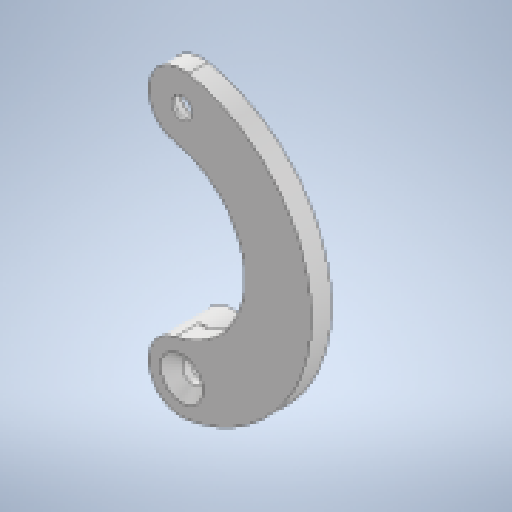
# Autodesk Inventor part: rotor_arm
Saved by Autodesk Inventor 2024 (Build 280153000, 153)
## iProperties
Created: 2025-06-26
Part Number: rotor_arm
Material: 一般
Document SubType Name: Modeling
Designer: kshau
Density: 1 g/cm^3
Appearance: 既定
Author: kshau
Autodesk Inventor part; units mm, degrees
ref_plane "YZ Plane" through (0, 0, 0) normal (1, 0, 0) x (0, 1, 0)
ref_plane "XZ Plane" through (0, 0, 0) normal (0, 1, 0) x (-1, 0, 0)
ref_plane "XY Plane" through (0, 0, 0) normal (0, 0, 1) x (1, 0, 0)
sketch "スケッチ1" plane through (0, 0, 0) normal (0, 0, 1) x (1, 0, 0)
  circle A0 centre (0, 0) radius 5
  circle A1 centre (0, 35) radius 5
  line L0 (0, 35) -> (0, 0)
  arc A2 (0.968731, -4.905258) -> (0.968731, 39.905258) centre (-3.456045, 17.5) ccw
  arc A3 (-0.968731, 4.905258) -> (-0.968731, 30.094742) centre (-3.456045, 17.5) ccw
  point P0 (0, 30)
  point P1 (0, 29.864061)
  point P2 (0, 5.135939)
  point P3 (0, 5)
  dimension "d0" = 10
  dimension "d1" = 10
  dimension "d2" = 35
  dimension "d3" = 22.838
  dimension "d4" = 12.838
  constraints: 8 point on circle, 4 centre point, 4 tangent, 2 end point, 1 coincident, 1 vertical
  measures "d0" diameter of A0
  measures "d1" diameter of A1
  measures "d2" distance of L0.end L0.start
  measures "d3" radius of A2
  measures "d4" radius of A3
extrude "押し出し1" add sketch "スケッチ1" along normal blind 3 contours A0 | A3 L0 A0 | A0 L0 A3 A1 A2 | A1 | A3 A1 L0
sketch "スケッチ2" plane through (0, 0, 0) normal (0, 0, -1) x (-1, 0, 0)
  circle A0 centre (0, 0) radius 5
  constraints: 1 centre point, 1 coincident
extrude "押し出し2" add sketch "スケッチ2" along normal blind 4.8
sketch "スケッチ3" plane through (0, 0, -4.8) normal (0, 0, -1) x (-1, 0, 0)
  circle A0 centre (0, 0) radius 3.1
  dimension "d9" = 6.2
  constraints: 1 centre point, 1 coincident
  measures "d9" diameter of A0
extrude "押し出し3" cut sketch "スケッチ3" against normal blind 5
sketch "スケッチ4" plane through (0, 0, 3) normal (0, 0, 1) x (1, 0, 0)
  circle A0 centre (0, 0) radius 3.1
  arc A1 (0.968731, 39.905258) -> (-0.968731, 30.094742) centre (0, 35) ccw
  point P0 (0, 30)
  constraints: 2 coincident
hole "穴1" at (0, 0, 3) at (0, 35, 3) direction (0, 0, -1) diameter 3.1 end through all
sketch "スケッチ5" plane through (0, 0, 0) normal (0, 0, -1) x (-1, 0, 0)
  circle A0 centre (0, 35) radius 1.55 projected
  circle A1 centre (0, 35) radius 3.1
  point P0 (0, 0)
  dimension "d19" = 6.2
  constraints: 1 centre point, 1 coincident
  measures "d19" diameter of A1
extrude "押し出し4" cut sketch "スケッチ5" against normal blind 2.5
sketch "スケッチ6" plane through (0, 0, 3) normal (0, 0, 1) x (1, 0, 0)
  circle A0 centre (0, 0) radius 1.55 projected
  constraints: 1 coincident
hole "穴2" at (0, 0, 3) direction (0, 0, -1) diameter 3.1 end through all countersink diameter 6.3 countersink angle 90
fillet "フィレット1" radius 0.5 3 edges at (3.1, 0, -4.8) (3.1, 35, 0) (4.9053, 0.9687, 0)
